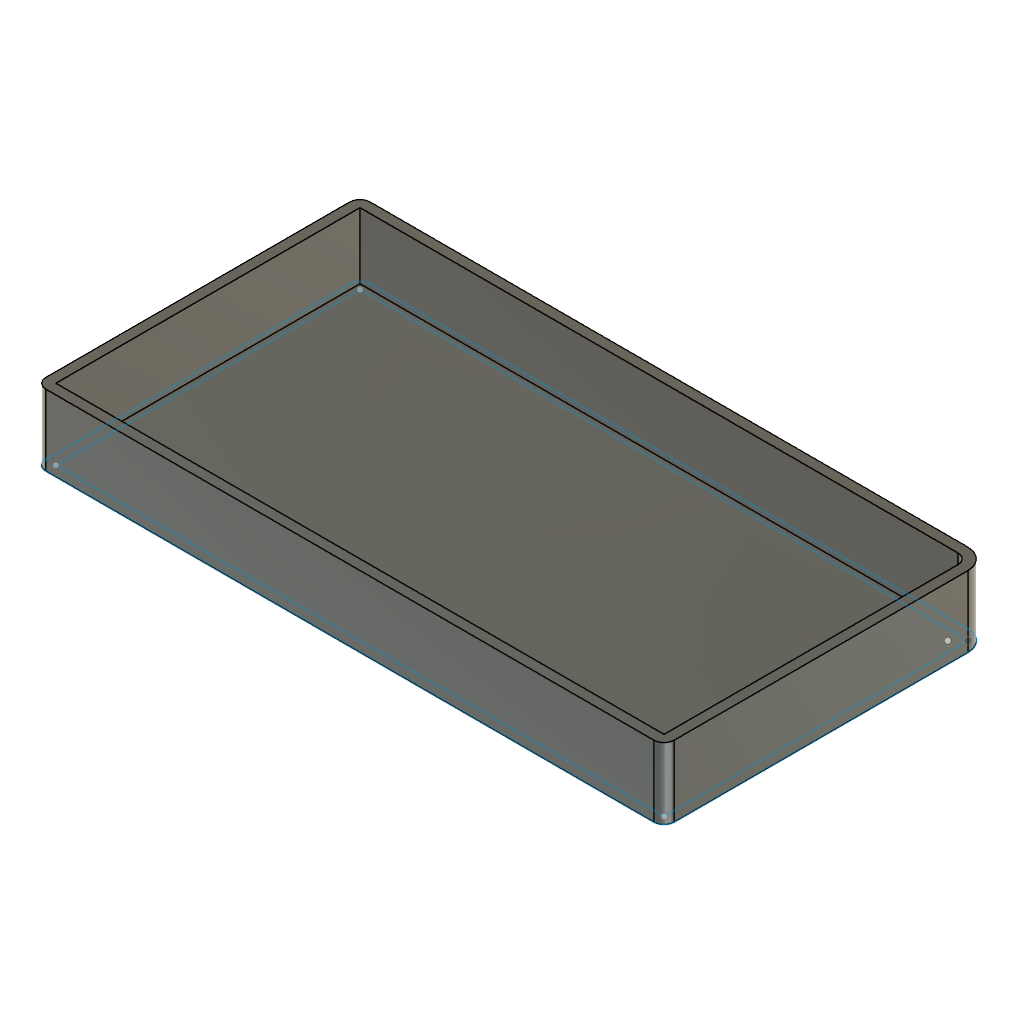
Draingaebox (Autodesk Fusion 360 design; units mm, degrees)
part number: 2026-09-20-23-00-51-797
Autodesk Fusion 360 part; units mm, degrees
sketch "Sketch1" plane through (0, 0, 0) normal (0, 0, 1) x (1, 0, 0)
  line L0 (-150, 40) -> (145, 40)
  line L1 (150, 35) -> (150, -110)
  line L2 (150, -110) -> (-150, -110)
  line L3 (-150, -110) -> (-150, 40)
  arc A0 (150, 35) -> (145, 40) centre (145, 35) ccw
  line L4 (155, 35) -> (155, -110)
  line L5 (150, -115) -> (-150, -115)
  line L6 (-155, -110) -> (-155, 40)
  line L7 (-150, 45) -> (145, 45)
  arc A1 (155, 35) -> (145, 45) centre (145, 35) ccw
  arc A2 (-150, 45) -> (-155, 40) centre (-150, 40) ccw
  arc A3 (-155, -110) -> (-150, -115) centre (-150, -110) ccw
  arc A4 (150, -115) -> (155, -110) centre (150, -110) ccw
  point P0 (150, 40)
  dimension "d1" = 300
  dimension "d2" = 150
  dimension "d4" = 5
  dimension "d5" = 5
  dimension "d6" = 5
  dimension "d7" = 5
  dimension "d8" = 5
  constraint perpendicular L0 L1
  constraint parallel L0 L2
  constraint parallel L1 L3
  constraint horizontal L0
  constraint coincident P0 L0
  constraint coincident P0 L1
  constraint tangent L0 A0
  constraint tangent L1 A0
  constraint concentric A0 A1
  constraint tangent L4 A1
  constraint tangent L7 A1
  constraint tangent L6 A2
  constraint tangent L7 A2
  constraint equal A0 A2
  constraint tangent L5 A3
  constraint tangent L6 A3
  constraint equal A0 A3
  constraint tangent L4 A4
  constraint tangent L5 A4
  constraint equal A0 A4
  measures "d1" distance of L0.start P0
  measures "d2" distance of L0.start L2.end
  measures "d4" radius of A0
  measures "d5" distance of L1 L4
  measures "d6" distance of L2 L5
  measures "d7" distance of L3 L6
  measures "d8" distance of L0 L7
extrude "Extrude1" add sketch "Sketch1" along normal blind 20
extrude "Extrude2" add sketch "Sketch1" along normal blind 2.5 contours L0 L1 L2 L3 A0
extrude "Extrude3" add 1 faces at (50, -111.6667, 20) along direction (0, 0, 1) blind 15
